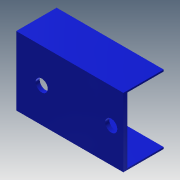
# Autodesk Inventor part: kolejnicka_ruka
Saved by Autodesk Inventor 2013 (Build 170138000, 138)
## iProperties
Created: 2013-03-23
Part Number: kolejnicka_ruka
Material: Generic
Document SubType Name: Modeling
Designer: idle-rug
Density: 1 g/cm^3
Author: idle-rug
Autodesk Inventor part; units mm, degrees
ref_plane "YZ Plane" through (0, 0, 0) normal (1, 0, 0) x (0, 1, 0)
ref_plane "XZ Plane" through (0, 0, 0) normal (0, 1, 0) x (-1, 0, 0)
ref_plane "XY Plane" through (0, 0, 0) normal (0, 0, 1) x (1, 0, 0)
sketch "Sketch1" plane through (0, 0, 0) normal (0, 1, 0) x (-1, 0, 0)
  line L0 (12.35, 8.5) -> (-12.35, 8.5)
  line L1 (-12.35, 8.5) -> (-12.35, -8.5)
  line L2 (-12.35, -8.5) -> (12.35, -8.5)
  line L3 (12.35, -8.5) -> (12.35, 8.5)
  line L4 (12.35, 8.5) -> (-12.35, -8.5) construction
  line L5 (-12.35, 8.5) -> (12.35, -8.5) construction
  point P0 (0, 0)
  dimension "d0" = 24.7
  dimension "d1" = 17
  constraints: 12 end point, 2 midpoint, 2 parallel, 1 horizontal, 1 perpendicular
  measures "d0" distance of L2.end L1.end
  measures "d1" distance of L1.end L0.end
extrude "Extrusion1" add sketch "Sketch1" along normal blind 10
sketch "Sketch2" plane through (0, 10, 0) normal (0, 1, 0) x (1, 0, 0)
  line L0 (-12.35, 8.1) -> (12.35, 8.1)
  line L1 (12.35, 8.1) -> (12.35, -8.1)
  line L2 (12.35, -8.1) -> (-12.35, -8.1)
  line L3 (-12.35, -8.1) -> (-12.35, 8.1)
  line L4 (-12.35, 8.1) -> (12.35, -8.1) construction
  line L5 (12.35, 8.1) -> (-12.35, -8.1) construction
  point P0 (0, 0)
  dimension "d4" = 24.7
  dimension "d5" = 16.2
  constraints: 12 end point, 2 midpoint, 2 parallel, 1 horizontal, 1 perpendicular
  measures "d4" distance of L1.end L2.end
  measures "d5" distance of L0.end L1.end
extrude "Extrusion2" cut sketch "Sketch2" against normal blind 9
sketch "Sketch3" plane through (0, 0, 0) normal (0, -1, 0) x (1, 0, 0)
  line L0 (-12.35, -8.5) -> (-12.35, 8.5) projected
  line L1 (12.35, 8.5) -> (12.35, -8.5) projected
  line L2 (-12.35, 0) -> (-9.35, 0)
  circle A0 centre (-9.35, 0) radius 1.5
  line L3 (12.35, 0) -> (9.35, 0)
  circle A1 centre (9.35, 0) radius 1.5
  point P0 (0, 0)
  dimension "d8" = 3
  dimension "d9" = 3
  dimension "d10" = 3
  dimension "d11" = 3
  constraints: 4 end point, 2 centre point, 2 coincident, 2 midpoint, 1 collinear, 1 perpendicular
  measures "d8" distance of L2.start L2.end
  measures "d9" diameter of A0
  measures "d10" distance of L3.start L3.end
  measures "d11" diameter of A1
extrude "Extrusion3" cut sketch "Sketch3" against normal blind 1
sketch "Sketch4" plane through (-12.35, 0, -8.5) normal (-1, 0, 0) x (0, 0, 1)
  line L0 (0.4, 1) -> (0.4, 10) projected
  line L1 (0, 10) -> (0.4, 10) projected
  line L2 (0, 0) -> (0, 10) projected
  line L3 (0, 0) -> (17, 0) projected
  line L4 (17, 0) -> (17, 10) projected
  line L5 (16.6, 10) -> (17, 10) projected
  line L6 (16.6, 10) -> (16.6, 1) projected
  line L7 (16.6, 1) -> (0.4, 1) projected
  point P0 (8.5, 0)
extrude "Extrusion4" add sketch "Sketch4" along normal blind 2
sketch "Sketch5" plane through (-14.35, 0, -8.5) normal (-1, 0, 0) x (0, 0, 1)
  line L0 (0.4, 1) -> (0.4, 10) projected
  line L1 (0.4, 10) -> (0, 10) projected
  line L2 (0, 10) -> (0, 0) projected
  line L3 (0, 0) -> (17, 0) projected
  line L4 (17, 0) -> (17, 10) projected
  line L5 (17, 10) -> (16.6, 10) projected
  line L6 (16.6, 10) -> (16.6, 1) projected
  line L7 (16.6, 1) -> (0.4, 1) projected
  point P0 (8.5, 0)
extrude "Extrusion5" cut sketch "Sketch5" against normal blind 0.2
sketch "Sketch6" plane through (0, 0, 0) normal (0, -1, 0) x (1, 0, 0)
  line L0 (-14.15, 8.5) -> (-14.15, -8.5) projected
  line L1 (-14.15, 8.5) -> (12.35, 8.5) projected
  circle A0 centre (-9.35, 0) radius 1.5 projected
  line L2 (-14.15, 0) -> (-12.15, 0)
  line L3 (-12.15, 0) -> (-10.15, 0)
  line L4 (-10.15, 0) -> (-7.15, 0)
  point P0 (0, 0)
  dimension "d18" = 2
  dimension "d19" = 2
  dimension "d20" = 3
  constraints: 6 end point, 2 collinear, 1 midpoint, 1 parallel
  measures "d18" distance of L2.start L2.end
  measures "d19" distance of L2.end L3.end
  measures "d20" distance of L3.end L4.end
extrude "Extrusion6" add sketch "Sketch6" against normal blind 1
sketch "Sketch7" plane through (0, 0, 0) normal (0, -1, 0) x (1, 0, 0)
  line L0 (-14.15, 8.5) -> (-14.15, -8.5) projected
  line L1 (-14.15, 8.5) -> (12.35, 8.5) projected
  line L2 (-14.15, 0) -> (-10.85, 0)
  line L3 (-10.85, 0) -> (-7.85, 0)
  circle A0 centre (-7.85, 0) radius 1.5
  point P0 (0, 0)
  dimension "d29" = 3.3
  dimension "d30" = 3
  dimension "d31" = 3
  constraints: 4 end point, 1 centre point, 1 coincident, 1 collinear, 1 midpoint, 1 parallel
  measures "d29" distance of L2.start L2.end
  measures "d30" distance of L2.end L3.end
  measures "d31" diameter of A0
extrude "Extrusion7" cut sketch "Sketch7" against normal blind 1
body "Solid1"
